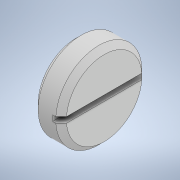
# Autodesk Inventor part: 711137
Saved by Autodesk Inventor 2022 (Build 260153000, 153)
## iProperties
Created: 2021-10-22
Part Number: 711137
Material: Типовые
Document SubType Name: Modeling
Designer: RaNSiD
Density: 1 g/cm^3
Appearance: По умолчанию
Author: RaNSiD
Autodesk Inventor part; units mm, degrees
ref_plane "YZ Plane" through (0, 0, 0) normal (1, 0, 0) x (0, 1, 0)
ref_plane "XZ Plane" through (0, 0, 0) normal (0, 1, 0) x (-1, 0, 0)
sketch "Эскиз1" plane through (0, 0, 0) normal (0, 0, 1) x (1, 0, 0)
  line L0 (0, 0) -> (0, 20)
  line L1 (0, 20) -> (2.8284, 22.8284)
  line L2 (0, 0) -> (15, 0)
  line L3 (15, 0) -> (15, 20)
  line L4 (15, 20) -> (12.1716, 22.8284)
  line L5 (12.1716, 22.8284) -> (2.8284, 22.8284)
  dimension "d0" = 20
  dimension "d1" = 4
  dimension "d2" = 135
  dimension "d3" = 15
  dimension "d4" = 4
  dimension "d5" = 135
  constraints: 12 end point, 1 horizontal, 1 parallel, 1 perpendicular, 1 vertical
  measures "d0" distance of L0.start L0.end
  measures "d1" distance of L0.end L1.end
  measures "d2" angle of L0 L1
  measures "d3" distance of L0.start L2.end
  measures "d4" distance of L3.end L4.end
  measures "d5" angle of L4 L3
revolve "Вращение1" add sketch "Эскиз1" angle 360 about axis through (0, 0, 0) along (1, 0, 0)
sketch "Эскиз2" plane through (0, 0, 0) normal (-1, 0, 0) x (0, 0, 1)
  point P0 (0, 0)
  point P1 (0, 18)
  point P2 (-15.5885, 9)
  point P3 (-15.5885, -9)
  point P4 (0, -18)
  point P5 (15.5885, -9)
  point P6 (15.5885, 9)
  dimension "d7" = 18
  dimension "d10" = 360
  constraints: 1 vertical alignment, 7 other
  measures "d7" distance of point (0, 0) point (0, 18)
hole "Отверстие1" at (0, 18, 0) at (0, 9, -15.5885) at (0, -9, -15.5885) at (0, -18, 0) at (0, -9, 15.5885) at (0, 9, 15.5885) direction (1, 0, 0) diameter 4 depth 4
sketch "Эскиз3" plane through (0, 0, 0) normal (0, 0, 1) x (1, 0, 0)
  line L0 (0, 0) -> (0, 8)
  line L1 (0, 8) -> (0.7, 7.3)
  line L2 (0, 8) -> (0.9899, 8) construction
  line L3 (0.7, 7.3) -> (6.643, 7.3)
  line L4 (6.643, 7.3) -> (6.643, 8)
  line L5 (6.643, 8) -> (7.343, 8)
  line L6 (7.343, 8) -> (7.343, 7.3)
  line L7 (7.343, 7.3) -> (10, 0)
  line L8 (10, 0) -> (0, 0)
  point P0 (0, 0)
  dimension "d19" = 45
  dimension "d20" = 70
  dimension "d21" = 8
  dimension "d22" = 0.7
  dimension "d23" = 0.7
  dimension "d24" = 10
  constraints: 18 end point, 5 perpendicular, 1 coincident, 1 equal length, 1 horizontal, 1 horizontal alignment, 1 point on line, 1 vertical alignment
  measures "d19" angle of L1 L2
  measures "d20" angle of L8 L7
  measures "d21" distance of L0.start L0.end
  measures "d22" distance of L5.end L6.end
  measures "d23" distance of L4.end L5.end
  measures "d24" distance of L7.end L0.start
revolve "Вращение2" cut sketch "Эскиз3" angle 360 about axis through (10, 0, 0) along (-1, 0, 0)
ref_plane "РабПлоскость1" through (0, 0, 30) normal (0, 0, 1) x (1, 0, 0)
sketch "Эскиз4" plane through (0, 0, 30) normal (0, 0, 1) x (1, 0, 0)
  line L0 (15, -20) -> (15, 20) construction
  line L1 (15, 1.5) -> (10.5, 1.5)
  line L2 (10.5, 1.5) -> (10.5, -1.5)
  line L3 (10.5, -1.5) -> (15, -1.5)
  line L4 (15, -1.5) -> (15, 1.5)
  point P0 (0, 0)
  point P1 (15, 0)
  point P2 (15, 0)
  dimension "d27" = 4.5
  dimension "d28" = 3
  constraints: 8 end point, 2 midpoint, 2 parallel, 1 coincident, 1 horizontal, 1 perpendicular, 1 point on line
  measures "d27" distance of L1.start L1.end
  measures "d28" distance of L1.end L2.end
extrude "Выдавливание1" cut sketch "Эскиз4" against normal through all
thread "Резьба1" size "M15x1.5" class "6H" standard "ANSI Metric M Profile" full length
